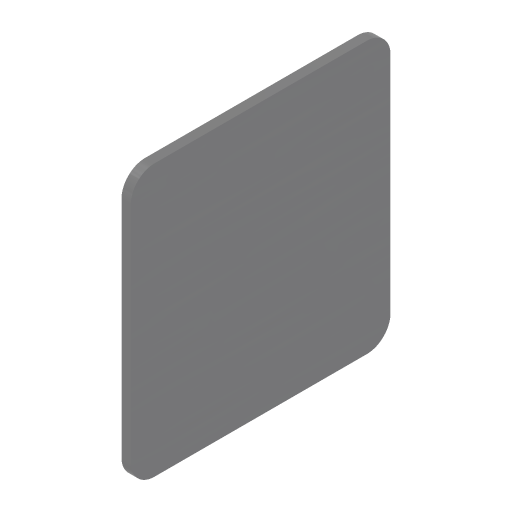
# Autodesk Inventor part: VIDRIO2
Saved by Autodesk Inventor 2024.1 (Build 281209000, 209)
## iProperties
Created: 2024-04-17
Part Number: VIDRIO2
Material: Glass
Document SubType Name: Modeling
Designer: Niler
Density: 2.18 g/cm^3
Appearance: Clear
Author: Niler
Autodesk Inventor part; units mm, degrees
ref_plane "YZ Plane" through (0, 0, 0) normal (1, 0, 0) x (0, 1, 0)
ref_plane "XZ Plane" through (0, 0, 0) normal (0, 1, 0) x (-1, 0, 0)
ref_plane "XY Plane" through (0, 0, 0) normal (0, 0, 1) x (1, 0, 0)
sketch "Sketch1" plane through (0, 0, 0) normal (1, 0, 0) x (0, 1, 0)
  line L0 (-95, 110) -> (95, 110)
  line L1 (115, 90) -> (115, -90)
  line L2 (95, -110) -> (-95, -110)
  line L3 (-115, -90) -> (-115, 90)
  line L4 (-115, 110) -> (115, -110) construction
  line L5 (115, 110) -> (-115, -110) construction
  arc A0 (115, 90) -> (95, 110) centre (95, 90) ccw
  arc A1 (95, -110) -> (115, -90) centre (95, -90) ccw
  arc A2 (-115, -90) -> (-95, -110) centre (-95, -90) ccw
  arc A3 (-95, 110) -> (-115, 90) centre (-95, 90) ccw
  point P0 (0, 0)
  dimension "d0" = 220
  dimension "d1" = 230
  dimension "d2" = 20
  constraints: 12 end point, 8 point on circle, 8 point on line, 8 tangent, 4 centre point, 3 equal radius, 2 midpoint, 2 parallel, 1 horizontal, 1 perpendicular
  measures "d0" distance between parallel lines of L2 L0
  measures "d1" distance between parallel lines of L3 L1
  measures "d2" radius of A0
extrude "Extrusion1" add sketch "Sketch1" along normal blind 8
body "Solid1"
